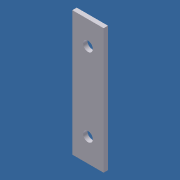
# Autodesk Inventor part: SM-M05
Saved by Autodesk Inventor 2012 SP1 (Build 160190100, 190)
## iProperties
Created: 2012-01-24
Part Number: SM-M05
Material: Steel, Mild
Document SubType Name: Modeling
Designer: ERF
Mass: 9.01616 g
Surface Area: 15.1613 cm^2
Volume: 1.14709 cm^3
Density: 7.86 g/cm^3
Description: Steel Flat Mending Bracket Zinc-Plated, 2" Length of Sides, 1/2" Width
Stock Number: 1394A31
Vendor: McMasterCarr
Project: Shapeoko
Author: ERF
Title: Belt Anchor
Autodesk Inventor part; units mm, degrees
ref_plane "YZ Plane" through (0, 0, 0) normal (1, 0, 0) x (0, 1, 0)
ref_plane "XZ Plane" through (0, 0, 0) normal (0, 1, 0) x (-1, 0, 0)
ref_plane "XY Plane" through (0, 0, 0) normal (0, 0, 1) x (1, 0, 0)
sketch "Sketch1" plane through (0, 0, 0) normal (0, 0, 1) x (1, 0, 0)
  line L0 (0, 50.8) -> (12.7, 50.8)
  line L1 (12.7, 50.8) -> (12.7, 0)
  line L2 (12.7, 0) -> (0, 0)
  line L3 (0, 0) -> (0, 50.8)
  dimension "d0" = 12.7
  dimension "d1" = 50.8
  constraints: 8 end point, 2 parallel, 1 horizontal, 1 perpendicular
  measures "d0" distance of L0.start L0.end
  measures "d1" distance of L0.end L1.end
extrude "Extrusion1" add sketch "Sketch1" along normal blind 1.778
sketch "Sketch2" plane through (0, 0, 1.778) normal (0, 0, 1) x (1, 0, 0)
  line L0 (12.7, 0) -> (0, 0) projected
  circle A0 centre (6.35, 9.525) radius 1.9844
  dimension "d4" = 3.9688
  dimension "d5" = 9.525
  constraints: 1 centre point
  measures "d4" diameter of A0
  measures "d5" distance from line of L0 A0.centre
extrude "Extrusion2" cut sketch "Sketch2" against normal through all
pattern_linear "Rectangular Pattern1" count 2 spacing 31.75 along (0, 1, 0) of "Extrusion2"
body "Solid1"
